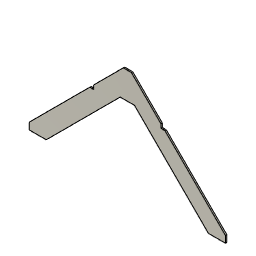
Arch (Autodesk Fusion 360 design; units mm, degrees)
Autodesk Fusion 360 part; units mm, degrees
sketch "Schizzo1" plane through (0, 0, 0) normal (0, 1, 0) x (1, 0, 0)
  line L0 (584, 0) -> (0, 0) construction
  line L1 (0, 0) -> (0, -20)
  line L2 (0, -20) -> (280, -300)
  line L3 (280, -300) -> (304, -300)
  line L4 (304, -300) -> (584, -20)
  line L5 (584, -20) -> (584, 0)
  line L6 (50.7107, 0) -> (270.7107, -220)
  line L7 (270.7107, -220) -> (313.2893, -220)
  line L8 (313.2893, -220) -> (533.2893, 0)
  line L9 (0, 0) -> (50.7107, 0)
  line L10 (533.2893, 0) -> (584, 0)
  line L11 (392.15, -211.85) -> (392.15, -200.15)
  line L12 (392.15, -200.15) -> (403.85, -200.15)
  line L13 (180.15, -200.15) -> (191.85, -200.15)
  line L14 (191.85, -200.15) -> (191.85, -211.85)
  line L15 (191.85, -200.15) -> (392.15, -200.15) construction
  dimension "d2" = 45
  dimension "d3" = 45
  dimension "d4" = 20
  dimension "d6" = 20
  dimension "d7" = 584
  dimension "d8" = 50
  dimension "d9" = 50
  dimension "d10" = 80
  dimension "d15" = 300
  dimension "d18" = 200.15
  dimension "d19" = 200.3
  dimension "d20" = 11.7
  constraint coincident L0.end L1.start
  constraint perpendicular L0 L1
  constraint perpendicular L1 L3
  constraint perpendicular L0 L5
  constraint vertical L1
  constraint coincident L0 L6.start
  constraint parallel L2 L6
  constraint parallel L0 L7
  constraint coincident L0 L8.end
  constraint perpendicular L6 L8
  constraint coincident L4 L11.start
  constraint vertical L11
  constraint coincident L4 L12.end
  constraint perpendicular L11 L12
  constraint coincident L2 L13.start
  constraint parallel L12 L13
  constraint coincident L2 L14.end
  constraint perpendicular L13 L14
  constraint perpendicular L11 L15
  constraint equal L12 L13
  measures "d2" angle of L2 L3
  measures "d3" angle of L3 L4
  measures "d4" distance of L0.start L4.end
  measures "d6" distance of L0.end L1.end
  measures "d7" distance of L0.start L0.end
  measures "d8" distance of L2 L6
  measures "d9" distance of L4 L8
  measures "d10" distance of L3 L7
  measures "d15" distance of L0 L3
  measures "d18" distance of L0 L15
  measures "d19" distance of L11.end L13.end
  measures "d20" distance of L13.start L13.end
extrude "Estrusione1" add sketch "Schizzo1" along normal blind 4 contours L1 L2 L3 L4 L5 L6 L7 L8 L9 L10 L11 L12 L13 L14
component "Component" placed x (1, 0, 0) y (0, 1, 0) z (0, 0, 1) at (0, 0, 0)
equation "d11 = h"
equation "h = 4 mm"
equation "t = 0.15 mm"
equation "d18 = 200 mm + t"
equation "d19 = 200 mm + 2 * t"
